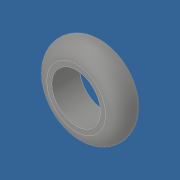
# Autodesk Inventor part: Wheel
Saved by Autodesk Inventor 2018 (Build 220112000, 112)
## iProperties
Created: 2018-02-14
Part Number: Wheel
Material: Rubber
Document SubType Name: Modeling
Designer: Cole
Density: 0.93 g/cm^3
Appearance: Smooth - Medium Gray
Author: Cole
Autodesk Inventor part; units mm, degrees
ref_plane "YZ Plane" through (0, 0, 0) normal (1, 0, 0) x (0, 1, 0)
ref_plane "XZ Plane" through (0, 0, 0) normal (0, 1, 0) x (-1, 0, 0)
ref_plane "XY Plane" through (0, 0, 0) normal (0, 0, 1) x (1, 0, 0)
sketch "Sketch1" plane through (0, 0, 0) normal (0, 0, 1) x (1, 0, 0)
  circle A0 centre (0, 0) radius 38.1
  dimension "d0" = 76.2
  constraints: 1 centre point, 1 coincident
  measures "d0" diameter of A0
extrude "Extrusion1" add sketch "Sketch1" along normal blind 24.384
full round fillet "Fillet1" first side at (18.352, 0, 24.384) centre faces at (37.9935, -2.8472, 16.256) second side at (18.352, 0, 0)
sketch "Sketch2" plane through (0, 0, 24.384) normal (0, 0, 1) x (1, 0, 0)
  circle A0 centre (0, 0) radius 21.4312
  dimension "d3" = 42.8625
  constraints: 1 centre point, 1 coincident
  measures "d3" diameter of A0
extrude "Extrusion2" cut sketch "Sketch2" against normal blind 24.384
body "Solid1"
